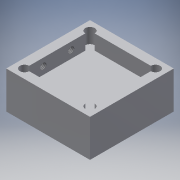
# Autodesk Inventor part: Large-cuvette-mount-40mm-V3
Saved by Autodesk Inventor 2016 (Build 200138000, 138)
## iProperties
Created: 2015-10-07
Part Number: Large-cuvette-mount-40mm-V3
Material: PC/ABS Plastic
Document SubType Name: Modeling
Designer: voigt
Density: 0.357273 g/cm^3
Appearance: Smooth - White
Author: voigt
Autodesk Inventor part; units mm, degrees
note: some values were not read from the file. Chosen so that the rebuilt part matches the saved one: direction of "Hole3".
ref_plane "YZ Plane" through (0, 0, 0) normal (1, 0, 0) x (0, 1, 0)
ref_plane "XZ Plane" through (0, 0, 0) normal (0, 1, 0) x (-1, 0, 0)
ref_plane "XY Plane" through (0, 0, 0) normal (0, 0, 1) x (1, 0, 0)
sketch "Sketch1" plane through (0, 0, 0) normal (0, 0, 1) x (1, 0, 0)
  line L0 (0, 31.5) -> (0, -31.5) construction
  line L1 (-31.5, 0) -> (31.5, 0) construction
  line L2 (-22.5, 22.5) -> (22.5, 22.5)
  line L3 (22.5, 22.5) -> (22.5, -22.5)
  line L4 (22.5, -22.5) -> (-22.5, -22.5)
  line L5 (-22.5, -22.5) -> (-22.5, 22.5)
  point P0 (0, 0)
  dimension "d0" = 45
  dimension "d1" = 45
  constraints: 8 end point, 2 parallel, 1 horizontal, 1 perpendicular, 2 other
  measures "d0" distance of L2.end L3.end
  measures "d1" distance of L3.end L4.end
extrude "Extrusion1" add sketch "Sketch1" along normal blind 20
sketch "Sketch4" plane through (0, 0, 20) normal (0, 0, 1) x (1, 0, 0)
  line L0 (-31.5, 0) -> (31.5, 0) construction
  line L1 (0, 31.5) -> (0, -31.5) construction
  line L2 (-17.575, 17.575) -> (17.575, 17.575) construction
  line L3 (17.575, 17.575) -> (17.575, -17.575) construction
  line L4 (17.575, -17.575) -> (-17.575, -17.575) construction
  line L5 (-17.575, -17.575) -> (-17.575, 17.575) construction
  point P0 (0, 0)
  dimension "d15" = 35.15
  dimension "d16" = 35.15
  constraints: 8 end point, 4 coincident, 2 parallel, 1 horizontal, 1 perpendicular, 2 other
  measures "d15" distance of L2.start L2.end
  measures "d16" distance of L4.end L2.start
hole "Hole2" at (-17.575, 17.575, 20) at (17.575, 17.575, 20) at (17.575, -17.575, 20) at (-17.575, -17.575, 20) at (-17.575, 17.575, 20) at (17.575, 17.575, 20) direction (0, 0, -1) diameter 5 depth 8
sketch "Sketch5" plane through (0, 0, 20) normal (0, 0, 1) x (1, 0, 0)
  circle A0 centre (-17.575, 17.575) radius 2.5 projected
  circle A1 centre (17.575, -17.575) radius 2.5 projected
  line L0 (-17.575, 17.575) -> (17.575, 17.575)
  line L1 (17.575, 17.575) -> (17.575, -17.575)
  line L2 (17.575, -17.575) -> (-17.575, -17.575)
  line L3 (-17.575, -17.575) -> (-17.575, 17.575)
  point P0 (0, 0)
  constraints: 8 end point, 2 parallel, 1 horizontal, 1 perpendicular
extrude "Extrusion3" cut sketch "Sketch5" against normal blind 8 contours L0 L1 A1 L2 L3 A0 | A0 L3 L0 | L1 L2 A1 picked at (-15.9292, 17.3896) picked at (17.028, -16.0118)
sketch "Sketch6" plane through (-22.5, -22.5, 0) normal (-1, 0, 0) x (0, 0, 1)
  line L0 (0, 45) -> (20, 45) projected
  line L1 (0, 0) -> (20, 0) projected
  line L2 (20, 7.425) -> (12, 7.425) construction
  line L3 (20, 37.575) -> (20, 7.425) construction
  line L4 (12, 37.575) -> (20, 37.575) construction
  line L5 (12, 7.425) -> (12, 37.575) construction
  line L6 (16, 37.575) -> (16, 7.425) construction
  point P0 (0, 22.5)
  point P1 (16, 30)
  point P2 (16, 15)
  dimension "d26" = 15
  dimension "d27" = 15
  constraints: 2 end point, 2 midpoint, 2 point on line
  measures "d26" distance from line of L1 point (16, 15)
  measures "d27" distance from line of L0 point (16, 30)
hole "Hole3" at (-22.5, 7.5, 16) at (-22.5, -7.5, 16) direction (1, 0, 0) diameter 3.242 end up to surface thread size "M4x0.7" class "6H" standard "ANSI Metric M Profile"
sketch "Sketch8" plane through (0, 0, 0) normal (0, 0, -1) x (-1, 0, 0)
  line L0 (22.5, 22.5) -> (-22.5, 22.5) construction
  line L1 (-22.5, 22.5) -> (-22.5, -22.5) construction
  line L2 (-22.5, -22.5) -> (22.5, -22.5) construction
  line L3 (22.5, -22.5) -> (22.5, 22.5) construction
  line L4 (0, -38.5) -> (0, 38.5) construction
  line L5 (-38.5, 0) -> (38.5, 0) construction
  line L6 (-12.5, -12.5) -> (12.5, -12.5)
  line L7 (12.5, -12.5) -> (12.5, 12.5)
  line L8 (12.5, 12.5) -> (-12.5, 12.5)
  line L9 (-12.5, 12.5) -> (-12.5, -12.5)
  point P0 (0, 0)
  dimension "d44" = 25
  dimension "d45" = 25
  constraints: 8 end point, 2 parallel, 1 horizontal, 1 perpendicular, 2 other
  measures "d44" distance of L6.start L6.end
  measures "d45" distance of L8.end L6.start
extrude "Extrusion4" cut sketch "Sketch8" against normal blind 6
sketch "Sketch9" plane through (0, 0, 0) normal (0, 0, -1) x (-1, 0, 0)
  line L0 (12.5, 12.5) -> (12.5, -12.5) construction
  line L1 (12.5, -12.5) -> (-12.5, -12.5) construction
  line L2 (-12.5, -12.5) -> (-12.5, 12.5) construction
  line L3 (-12.5, 12.5) -> (12.5, 12.5) construction
  line L4 (22.5, 22.5) -> (-22.5, 22.5) construction
  line L5 (-22.5, 22.5) -> (-22.5, -22.5) construction
  line L6 (-22.5, -22.5) -> (22.5, -22.5) construction
  line L7 (22.5, -22.5) -> (22.5, 22.5) construction
  line L8 (12.5, -12.5) -> (-12.5, -12.5) construction
  point P0 (0, 0)
  constraints: 4 coincident
hole "Hole5" at (-12.5, 12.5, 0) at (-12.5, -12.5, 0) at (12.5, -12.5, 0) at (12.5, 12.5, 0) direction (0, 0, 1) diameter 3 depth 6
sketch "Sketch10" plane through (0, 0, 6) normal (0, 0, -1) x (-1, 0, 0)
  point P0 (0, 0)
  point P1 (0, 0)
  constraints: 1 coincident
hole "Hole6" at (0, 0, 6) direction (0, 0, 1) diameter 3.242 depth 4 tip angle 118 thread size "M4x0.7" class "6H" standard "ANSI Metric M Profile"
body "Solid1"
